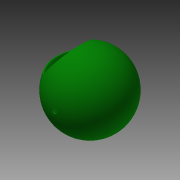
# Autodesk Inventor part: ping pong ball
Saved by Autodesk Inventor 2013 (Build 170138000, 138)
## iProperties
Created: 2012-09-25
Part Number: ping pong ball
Material: Generic
Document SubType Name: Modeling
Designer: uqgtayle
Density: 1 g/cm^3
Author: uqgtayle
Autodesk Inventor part; units mm, degrees
sketch "Sketch1" plane through (0, 0, 0) normal (0, 0, 1) x (1, 0, 0)
  line L0 (15.9491, 0) -> (16.0494, 0)
  line L1 (-19.8, 0) -> (19.8, 0)
  arc A0 (19.8, 0) -> (-19.8, 0) centre (0, 0) ccw
  dimension "d32" = 39.6
  constraints: 4 end point, 2 point on circle, 1 centre point, 1 coincident, 1 collinear, 1 horizontal, 1 point on line
  measures "d32" diameter of A0
ref_plane "Work Plane1" through (0, 0, 7) normal (0, 0, 1) x (1, 0, 0)
revolve "Revolution3" add sketch "Sketch1" angle 360 about axis through (15.9491, 0, 0) along (1, 0, 0)
ref_plane "Work Plane2" through (0, 0, 11) normal (0, 0, 1) x (1, 0, 0)
sketch "Sketch17" plane through (0, 0, 0) normal (0, 1, 0) x (-1, 0, 0)
  line L0 (26.807, 7) -> (13.1257, 7)
  line L1 (13.1257, 7) -> (3.4348, 21.8215)
  line L2 (3.4348, 21.8215) -> (26.807, 7)
  point P0 (0, 0)
  dimension "d50" = 7
  constraints: 6 end point, 1 horizontal
  measures "d50" distance from line of L0 point (0, 0)
extrude "Extrusion10" cut sketch "Sketch17" along normal through all both and the other way through all
shell "Shell4" thickness 0.5 removed faces 2 at (-15.7431, -1.7688, 7) at (-10.8801, -4.3558, 10.4345)
sketch "Sketch16" plane through (0, 0, 0) normal (0, 1, 0) x (-1, 0, 0)
  circle A0 centre (0, 0) radius 1.55
  dimension "d39" = 3.1
  constraints: 1 centre point, 1 coincident
  measures "d39" diameter of A0
extrude "Extrusion9" cut sketch "Sketch16" along normal through all both and the other way through all
sketch "Sketch18" plane through (0, 0, 0) normal (1, 0, 0) x (0, 1, 0)
  circle A0 centre (0, 0) radius 1
  dimension "d46" = 2
  constraints: 1 centre point, 1 coincident
  measures "d46" diameter of A0
extrude "Extrusion11" cut sketch "Sketch18" against normal through all
ref_plane "Work Plane3" through (0, 0, -20.5) normal (0, 0, 1) x (1, 0, 0)
body "Solid3"
